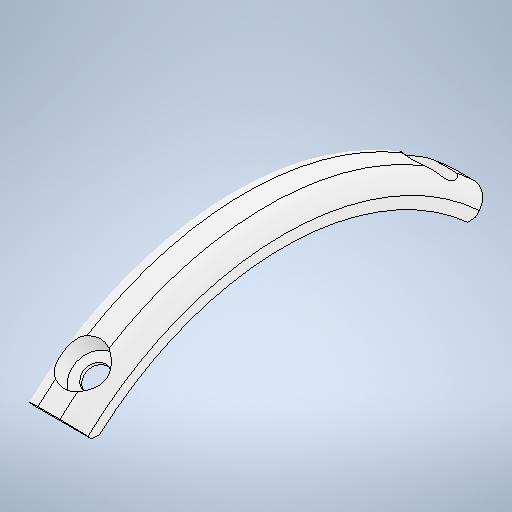
# Autodesk Inventor part: joint3_frame_support_fixture
Saved by Autodesk Inventor 2025.3 (Build 293356030, 356C)
## iProperties
Created: 2025-11-26
Part Number: joint3_frame_support_fixture
Material: PLA filament
Document SubType Name: Modeling
Designer: MSI
Mass: 3.8013 g
Surface Area: 23.8298 cm^2
Volume: 3.16775 cm^3
Density: 1.2 g/cm^3
Appearance: 일반
Author: MSI
Autodesk Inventor part; units mm, degrees
ref_plane "YZ Plane" through (0, 0, 0) normal (1, 0, 0) x (0, 1, 0)
ref_plane "XZ Plane" through (0, 0, 0) normal (0, 1, 0) x (-1, 0, 0)
ref_plane "XY Plane" through (0, 0, 0) normal (0, 0, 1) x (1, 0, 0)
sketch "스케치1" plane through (0, 0, 0) normal (1, 0, 0) x (0, 1, 0)
  circle A0 centre (0, 0) radius 55
  line L0 (40.2245, 37.5099) -> (0, 0)
  line L1 (0, 0) -> (40.2245, -37.5099)
  line L2 (0, 0) -> (55, 0) construction
  circle A1 centre (0, 0) radius 50
  point P0 (36.5677, -34.0999)
  point P1 (36.5677, 34.0999)
  dimension "d0" = 110
  dimension "d1" = 43
  dimension "d2" = 43
  dimension "d3" = 5
  constraints: 6 end point, 3 point on circle, 2 centre point, 1 coincident, 1 horizontal
  measures "d0" diameter of A0
  measures "d1" angle of L2 L0
  measures "d2" angle of L2 L1
  measures "d3" radial gap between concentric circles of A0 A1
extrude "돌출1" add sketch "스케치1" along normal mid plane 10 contours A0 L1 A1 L0 picked at (41.1024, 33.6529)
sketch "스케치2" plane through (0, 0, 0) normal (1, 0, 0) x (0, 1, 0)
  line L0 (45.0996, 31.5791) -> (0, 0) construction
  line L1 (0, 0) -> (55, 0) construction
  arc A0 (40.2245, -37.5099) -> (40.2245, 37.5099) centre (0, 0) ccw projected
  dimension "d10" = 35
  constraints: 4 end point, 1 horizontal, 1 point on circle
  measures "d10" angle of L1 L0
ref_plane "작업 평면1" through (0, 45.0996, 31.5791) normal (0, -0.819152, -0.5735764) x (1, 0, 0)
sketch "스케치3" plane through (0, 45.0996, 31.5791) normal (0, -0.819152, -0.5735764) x (1, 0, 0)
  point P0 (0, 0)
  point P1 (0, 0)
  constraints: 1 coincident
hole "구멍1" at (0, 45.0996, 31.5791) direction (0, -0.819152, -0.5735764) diameter 4.5 end through all counterbore diameter 8 counterbore depth 4.4 clearance for "Socket Head Cap Screw ISO 4762" size "M4" standard "ISO"
mirror "미러1" about plane through (0, 0, 0) normal (0, 0, 1) of "구멍1"
fillet "모깎기1" radius 3 2 edges at (-5, 55, 0) (5, 55, 0)
chamfer "모따기1" distance 1 angle 45 2 edges at (0, 36.5677, 34.0999) (0, 36.5677, -34.0999)
equation "\"d2\" = d1"
